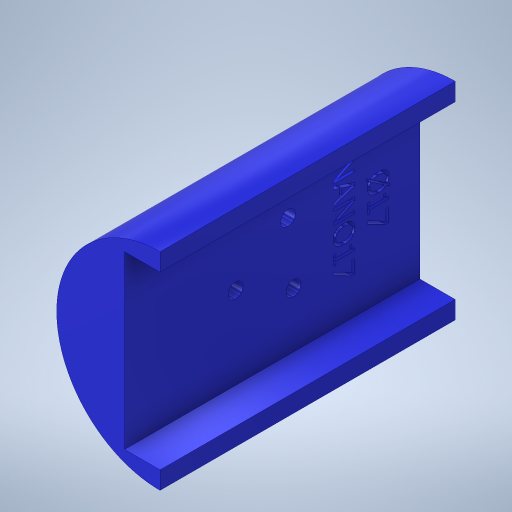
# Autodesk Inventor part: NANO17Shell18_A
Saved by Autodesk Inventor 2023 (Build 270158000, 158)
## iProperties
Created: 2016-07-01
Part Number: NANO17Shell18_A
Material: ABS Plastic
Document SubType Name: Modeling
Designer: Administrateur
Density: 1.06 g/cm^3
Appearance: Blue - Wall Paint - Glossy
Author: Administrateur
Autodesk Inventor part; units mm, degrees
ref_plane "XZ Plane" through (0, 0, 0) normal (0, 1, 0) x (-1, 0, 0)
sketch "Sketch1" plane through (0, 0, 0) normal (0, 0, 1) x (1, 0, 0)
  arc A0 (0, 17.5) -> (0, -17.5) centre (0, 0) ccw
  line L0 (0, 17.5) -> (0, 14.5)
  line L1 (0, 14.5) -> (-6, 14.5)
  line L2 (-6, 14.5) -> (-6, 0)
  line L3 (-46.5484, 0) -> (26.4312, 0) construction
  line L4 (0, -17.5) -> (0, -14.5)
  line L5 (0, -14.5) -> (-6, -14.5)
  line L6 (-6, -14.5) -> (-6, 0)
  dimension "d2" = 17.5
  dimension "d3" = 29
  dimension "d4" = 6
  dimension "d27" = 14.5
  dimension "d28" = 3
  constraints: 14 end point, 2 horizontal, 2 point on circle, 2 symmetric about line, 1 centre point, 1 coincident, 1 perpendicular, 1 vertical
  measures "d2" radius of A0
  measures "d3" distance between parallel lines of L5 L1
  measures "d4" distance of L0.end L1.end
  measures "d27" distance of L1.end L2.end
  measures "d28" distance of L0.start L0.end
extrude "Extrusion1" add sketch "Sketch1" along normal blind 50
sketch "Sketch2" plane through (-6, -14.5, 0) normal (1, 0, 0) x (0, 0, -1)
  line L0 (-25, 14.5) -> (-50, 14.5) construction
  line L1 (-50, 32) -> (-50, -3) construction
  line L2 (0, 32) -> (-50, 32) construction
  line L3 (-25, 32) -> (-25, -3) construction
  line L4 (0, -3) -> (-50, -3) construction
  circle A0 centre (-25, 14.5) radius 6.25 construction
  line L5 (-25, 14.5) -> (-22.3586, 20.1644) construction
  line L6 (-25, 14.5) -> (-31.2262, 13.9553) construction
  line L7 (-25, 14.5) -> (-21.4151, 9.3803) construction
  point P0 (0, 14.5)
  dimension "d6" = 12.5
  dimension "d7" = 115
  dimension "d10" = 360
  constraints: 10 end point, 4 coincident, 4 midpoint, 13 other
  measures "d7" angle of L0 L5
hole "Hole1" at (-6, -0.5447, 31.2262) at (-6, -5.1197, 21.4151) at (-6, 5.6644, 22.3586) direction (-1, 0, 0) diameter 2.5 end through all
ref_plane "Work Plane1" through (-17.5, 0, 0) normal (1, 0, 0) x (0, 1, 0)
sketch "Sketch3" plane through (-17.5, 0, 0) normal (1, 0, 0) x (0, 1, 0)
  line L0 (17.5, 0) -> (-17.5, 0) projected
  line L1 (-17.5, 0) -> (-17.5, 50) projected
  line L2 (17.5, 50) -> (-17.5, 50) projected
  line L3 (17.5, 0) -> (17.5, 50) projected
  circle A0 centre (5.6644, 22.3586) radius 1.25 projected
  circle A1 centre (-5.1197, 21.4151) radius 1.25 projected
  line L4 (5.6644, 22.3586) -> (-5.1197, 21.4151) construction
  circle A2 centre (-0.5447, 31.2262) radius 1.25 projected
  line L5 (-5.1197, 21.4151) -> (-0.5447, 31.2262) construction
  line L6 (-0.5447, 31.2262) -> (5.6644, 22.3586) construction
  point P0 (0, 0)
  point P1 (5.6644, 22.3586)
  point P2 (-5.1197, 21.4151)
  point P3 (-0.5447, 31.2262)
  constraints: 6 end point, 3 coincident, 3 horizontal alignment, 3 other
ref_plane "Work Plane2" through (-10, 0, 0) normal (1, 0, 0) x (0, 1, 0)
hole "Hole2" at (-17.5, 5.6644, 22.3586) at (-17.5, -5.1197, 21.4151) at (-17.5, -0.5447, 31.2262) direction (1, 0, 0) diameter 5 depth 7.5
sketch "Esquisse4" plane through (-6, -14.5, 0) normal (1, 0, 0) x (0, 0, -1)
  line L0 (-5.1227, 22.9938) -> (-5.1227, 7.2268) construction
  line L1 (-5.1227, 7.2268) -> (-14.5385, 7.2268) construction
  line L2 (-14.5385, 7.2268) -> (-14.5385, 22.9938) construction
  line L3 (-14.5385, 22.9938) -> (-5.1227, 22.9938) construction
  spline S0 degree 2 poles (-7.0883, 16.1895) (-7.9562, 16.1895) (-8.912, 17.0347) (-8.912, 17.7381) knots 0 0 0 1 2 2 2
  spline S1 degree 2 poles (-8.912, 17.7381) (-8.912, 17.9962) (-8.7759, 18.4415) (-8.6511, 18.6202) knots 0 0 0 1 2 2 2
  line L4 (-8.6511, 18.6202) -> (-9.1106, 18.9322)
  line L5 (-9.1106, 18.9322) -> (-9.1106, 19.2782)
  line L6 (-9.1106, 19.2782) -> (-8.4582, 18.8358)
  spline S2 degree 2 poles (-8.4582, 18.8358) (-8.2256, 19.0457) (-7.5392, 19.2839) (-7.0883, 19.2839) knots 0 0 0 1 2 2 2
  spline S3 degree 2 poles (-7.0883, 19.2839) (-6.2232, 19.2839) (-5.2645, 18.4359) (-5.2645, 17.7381) knots 0 0 0 1 2 2 2
  spline S4 degree 2 poles (-5.2645, 17.7381) (-5.2645, 17.4687) (-5.395, 17.0489) (-5.5226, 16.8617) knots 0 0 0 1 2 2 2
  line L7 (-5.5226, 16.8617) -> (-5.1227, 16.5923)
  line L8 (-5.1227, 16.5923) -> (-5.1227, 16.2434)
  line L9 (-5.1227, 16.2434) -> (-5.7127, 16.6461)
  spline S5 degree 2 poles (-5.7127, 16.6461) (-5.9452, 16.4306) (-6.6203, 16.1895) (-7.0883, 16.1895) knots 0 0 0 1 2 2 2
  spline S6 degree 2 poles (-7.0883, 16.6688) (-6.7649, 16.6688) (-6.2572, 16.7993) (-6.0899, 16.9071) knots 0 0 0 1 2 2 2
  line L10 (-6.0899, 16.9071) -> (-8.2937, 18.382)
  spline S7 degree 2 poles (-8.2937, 18.382) (-8.4015, 18.2487) (-8.5093, 17.948) (-8.5093, 17.7353) knots 0 0 0 1 2 2 2
  spline S8 degree 2 poles (-8.5093, 17.7353) (-8.5093, 17.2503) (-7.7775, 16.6688) (-7.0883, 16.6688) knots 0 0 0 1 2 2 2
  spline S9 degree 2 poles (-5.8772, 17.1) (-5.7722, 17.2219) (-5.6673, 17.5424) (-5.6673, 17.7353) knots 0 0 0 1 2 2 2
  spline S10 degree 2 poles (-5.6673, 17.7353) (-5.6673, 18.2231) (-6.3905, 18.8046) (-7.0883, 18.8046) knots 0 0 0 1 2 2 2
  spline S11 degree 2 poles (-7.0883, 18.8046) (-7.4059, 18.8046) (-7.8995, 18.6826) (-8.0753, 18.572) knots 0 0 0 1 2 2 2
  line L11 (-8.0753, 18.572) -> (-5.8772, 17.1)
  line L12 (-8.8383, 13.7957) -> (-8.8383, 15.5031)
  line L13 (-8.8383, 15.5031) -> (-8.4809, 15.5031)
  line L14 (-8.4809, 15.5031) -> (-8.4809, 14.8678)
  line L15 (-8.4809, 14.8678) -> (-6.1353, 14.8678)
  line L16 (-6.1353, 14.8678) -> (-6.1353, 15.5031)
  line L17 (-6.1353, 15.5031) -> (-5.8148, 15.5031)
  spline S12 degree 2 poles (-5.8148, 15.5031) (-5.8148, 15.1429) (-5.6106, 14.8026) (-5.3269, 14.7799) knots 0 0 0 1 2 2 2
  line L18 (-5.3269, 14.7799) -> (-5.3269, 14.4168)
  line L19 (-5.3269, 14.4168) -> (-8.4809, 14.4168)
  line L20 (-8.4809, 14.4168) -> (-8.4809, 13.7957)
  line L21 (-8.4809, 13.7957) -> (-8.8383, 13.7957)
  line L22 (-5.863, 10.9537) -> (-8.8383, 12.4683)
  line L23 (-8.8383, 12.4683) -> (-8.8383, 12.9675)
  line L24 (-8.8383, 12.9675) -> (-5.7495, 11.3678)
  line L25 (-5.7495, 11.3678) -> (-5.7495, 13.1745)
  line L26 (-5.7495, 13.1745) -> (-5.3383, 13.1745)
  line L27 (-5.3383, 13.1745) -> (-5.3383, 10.9537)
  line L28 (-5.3383, 10.9537) -> (-5.863, 10.9537)
  line L29 (-14.6009, 21.2381) -> (-14.6009, 21.76)
  line L30 (-14.6009, 21.76) -> (-11.5831, 23.3086)
  line L31 (-11.5831, 23.3086) -> (-14.6009, 23.3086)
  line L32 (-14.6009, 23.3086) -> (-14.6009, 23.7426)
  line L33 (-14.6009, 23.7426) -> (-11.1009, 23.7426)
  line L34 (-11.1009, 23.7426) -> (-11.1009, 23.0817)
  line L35 (-11.1009, 23.0817) -> (-13.872, 21.6721)
  line L36 (-13.872, 21.6721) -> (-11.1009, 21.6721)
  line L37 (-11.1009, 21.6721) -> (-11.1009, 21.2381)
  line L38 (-11.1009, 21.2381) -> (-14.6009, 21.2381)
  line L39 (-14.6009, 20.9063) -> (-11.1009, 19.7264)
  line L40 (-11.1009, 19.7264) -> (-11.1009, 19.1534)
  line L41 (-11.1009, 19.1534) -> (-14.6009, 17.9735)
  line L42 (-14.6009, 17.9735) -> (-14.6009, 18.4642)
  line L43 (-14.6009, 18.4642) -> (-13.6224, 18.7819)
  line L44 (-13.6224, 18.7819) -> (-13.6224, 20.1178)
  line L45 (-13.6224, 20.1178) -> (-14.6009, 20.4355)
  line L46 (-14.6009, 20.4355) -> (-14.6009, 20.9063)
  line L47 (-13.2253, 18.9095) -> (-11.5774, 19.4513)
  line L48 (-11.5774, 19.4513) -> (-13.2253, 19.9902)
  line L49 (-13.2253, 19.9902) -> (-13.2253, 18.9095)
  line L50 (-14.6009, 15.1372) -> (-14.6009, 15.6591)
  line L51 (-14.6009, 15.6591) -> (-11.5831, 17.2077)
  line L52 (-11.5831, 17.2077) -> (-14.6009, 17.2077)
  line L53 (-14.6009, 17.2077) -> (-14.6009, 17.6417)
  line L54 (-14.6009, 17.6417) -> (-11.1009, 17.6417)
  line L55 (-11.1009, 17.6417) -> (-11.1009, 16.9808)
  line L56 (-11.1009, 16.9808) -> (-13.872, 15.5712)
  line L57 (-13.872, 15.5712) -> (-11.1009, 15.5712)
  line L58 (-11.1009, 15.5712) -> (-11.1009, 15.1372)
  line L59 (-11.1009, 15.1372) -> (-14.6009, 15.1372)
  spline S13 degree 2 poles (-11.5008, 11.9521) (-11.7334, 11.7535) (-12.4141, 11.5323) (-12.8509, 11.5323) knots 0 0 0 1 2 2 2
  spline S14 degree 2 poles (-12.8509, 11.5323) (-13.2764, 11.5323) (-13.9656, 11.7479) (-14.1982, 11.9521) knots 0 0 0 1 2 2 2
  spline S15 degree 2 poles (-14.1982, 11.9521) (-14.4421, 12.1676) (-14.6747, 12.7377) (-14.6747, 13.0809) knots 0 0 0 1 2 2 2
  spline S16 degree 2 poles (-14.6747, 13.0809) (-14.6747, 13.4355) (-14.4336, 14.0027) (-14.1982, 14.2098) knots 0 0 0 1 2 2 2
  spline S17 degree 2 poles (-14.1982, 14.2098) (-13.9656, 14.4111) (-13.282, 14.6267) (-12.8509, 14.6267) knots 0 0 0 1 2 2 2
  spline S18 degree 2 poles (-12.8509, 14.6267) (-12.4113, 14.6267) (-11.7419, 14.4083) (-11.5008, 14.2069) knots 0 0 0 1 2 2 2
  spline S19 degree 2 poles (-11.5008, 14.2069) (-11.2683, 14.0027) (-11.0272, 13.4326) (-11.0272, 13.0809) knots 0 0 0 1 2 2 2
  spline S20 degree 2 poles (-11.0272, 13.0809) (-11.0272, 12.7235) (-11.2768, 12.1506) (-11.5008, 11.9521) knots 0 0 0 1 2 2 2
  spline S21 degree 2 poles (-12.8509, 12.0173) (-12.5049, 12.0173) (-11.9688, 12.1676) (-11.793, 12.3038) knots 0 0 0 1 2 2 2
  spline S22 degree 2 poles (-11.793, 12.3038) (-11.6115, 12.4427) (-11.4299, 12.8342) (-11.4299, 13.0781) knots 0 0 0 1 2 2 2
  spline S23 degree 2 poles (-11.4299, 13.0781) (-11.4299, 13.3305) (-11.6058, 13.7106) (-11.793, 13.8552) knots 0 0 0 1 2 2 2
  spline S24 degree 2 poles (-11.793, 13.8552) (-11.9717, 13.9942) (-12.5106, 14.1417) (-12.8509, 14.1417) knots 0 0 0 1 2 2 2
  spline S25 degree 2 poles (-12.8509, 14.1417) (-13.5402, 14.1417) (-14.2719, 13.5631) (-14.2719, 13.0781) knots 0 0 0 1 2 2 2
  spline S26 degree 2 poles (-14.2719, 13.0781) (-14.2719, 12.5931) (-13.5402, 12.0173) (-12.8509, 12.0173) knots 0 0 0 1 2 2 2
  line L60 (-14.6009, 9.1385) -> (-14.6009, 10.8459)
  line L61 (-14.6009, 10.8459) -> (-14.2436, 10.8459)
  line L62 (-14.2436, 10.8459) -> (-14.2436, 10.2106)
  line L63 (-14.2436, 10.2106) -> (-11.8979, 10.2106)
  line L64 (-11.8979, 10.2106) -> (-11.8979, 10.8459)
  line L65 (-11.8979, 10.8459) -> (-11.5774, 10.8459)
  spline S27 degree 2 poles (-11.5774, 10.8459) (-11.5774, 10.4857) (-11.3732, 10.1453) (-11.0896, 10.1226) knots 0 0 0 1 2 2 2
  line L66 (-11.0896, 10.1226) -> (-11.0896, 9.7596)
  line L67 (-11.0896, 9.7596) -> (-14.2436, 9.7596)
  line L68 (-14.2436, 9.7596) -> (-14.2436, 9.1385)
  line L69 (-14.2436, 9.1385) -> (-14.6009, 9.1385)
  line L70 (-11.6256, 6.2965) -> (-14.6009, 7.8111)
  line L71 (-14.6009, 7.8111) -> (-14.6009, 8.3102)
  line L72 (-14.6009, 8.3102) -> (-11.5122, 6.7106)
  line L73 (-11.5122, 6.7106) -> (-11.5122, 8.5173)
  line L74 (-11.5122, 8.5173) -> (-11.1009, 8.5173)
  line L75 (-11.1009, 8.5173) -> (-11.1009, 6.2965)
  line L76 (-11.1009, 6.2965) -> (-11.6256, 6.2965)
  point P0 (0, 14.5)
  constraints: 2 other
extrude "Extrusion2" cut sketch "Esquisse4" against normal blind 1
equation "\"d27\" = 0.5 * d3"
equation "\"d28\" = -0.5 * d3 + d2"
body "Solid1"
